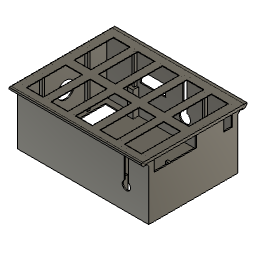
matek_enclosure (Autodesk Fusion 360 design; units mm, degrees)
Autodesk Fusion 360 part; units mm, degrees
note: some values were not read from the file. Set by a fixed rule: which sketch regions a step uses.
sketch "Sketch1" plane through (0, 0, 0) normal (0, 0, 1) x (1, 0, 0)
  line L0 (0, 0) -> (44, 0)
  line L1 (44, 0) -> (44, 29)
  line L2 (44, 29) -> (0, 29)
  line L3 (0, 29) -> (0, 0)
  line L4 (45, -1) -> (45, 30)
  line L5 (45, 30) -> (-1, 30)
  line L6 (-1, 30) -> (-1, -1)
  line L7 (-1, -1) -> (45, -1)
  line L8 (45.4, -1.4) -> (45.4, 30.4)
  line L9 (45.4, 30.4) -> (-1.4, 30.4)
  line L10 (-1.4, 30.4) -> (-1.4, -1.4)
  line L11 (-1.4, -1.4) -> (45.4, -1.4)
  line L12 (9, 30) -> (9, 29)
  line L13 (-1, 23) -> (0, 23)
  line L14 (9.8, 30) -> (9.8, 29)
  line L15 (-1, 22.2) -> (0, 22.2)
  line L16 (34.2, 30) -> (34.2, 29)
  line L17 (35, 30) -> (35, 29)
  line L18 (44, 23) -> (45, 23)
  line L19 (44, 22.2) -> (45, 22.2)
  line L20 (44, 6.8) -> (45, 6.8)
  line L21 (44, 6) -> (45, 6)
  line L22 (35, 0) -> (35, -1)
  line L23 (34.2, 0) -> (34.2, -1)
  line L24 (9, 0) -> (9, -1)
  line L25 (9.8, 0) -> (9.8, -1)
  line L26 (-1, 6.8) -> (0, 6.8)
  line L27 (-1, 6) -> (0, 6)
  line L28 (33.6, 30) -> (35.6, 30)
  line L29 (35.6, 30) -> (35.6, 28)
  line L30 (35.6, 28) -> (33.6, 28)
  line L31 (33.6, 28) -> (33.6, 30)
  line L32 (8.4, 30) -> (10.4, 30)
  line L33 (10.4, 30) -> (10.4, 28)
  line L34 (10.4, 28) -> (8.4, 28)
  line L35 (8.4, 28) -> (8.4, 30)
  line L36 (33.6, -1) -> (35.6, -1)
  line L37 (35.6, -1) -> (35.6, 1)
  line L38 (35.6, 1) -> (33.6, 1)
  line L39 (33.6, 1) -> (33.6, -1)
  line L40 (8.4, -1) -> (10.4, -1)
  line L41 (10.4, -1) -> (10.4, 1)
  line L42 (10.4, 1) -> (8.4, 1)
  line L43 (8.4, 1) -> (8.4, -1)
  dimension "d1" = 29
  dimension "d2" = 44
  dimension "d3" = 1
  dimension "d4" = 1.4
  dimension "d5" = 9
  dimension "d6" = 0.8
  dimension "d7" = 9
  dimension "d8" = 0.8
  dimension "d9" = 6
  dimension "d10" = 0.8
  dimension "d11" = 6
  dimension "d12" = 0.8
  dimension "d13" = 9
  dimension "d14" = 0.8
  dimension "d15" = 6
  dimension "d16" = 0.8
  dimension "d17" = 6
  dimension "d18" = 0.8
  dimension "d19" = 9
  dimension "d20" = 0.8
  dimension "d64" = 2
  dimension "d65" = 2
  dimension "d66" = 0.6
  dimension "d67" = 2
  dimension "d68" = 2
  dimension "d69" = 0.6
  dimension "d70" = 2
  dimension "d71" = 2
  dimension "d72" = 0.6
  dimension "d73" = 2
  dimension "d74" = 2
  dimension "d75" = 0.6
  constraint horizontal L0
  constraint vertical L1
  constraint horizontal L2
  constraint vertical L3
  constraint coincident L0.start L3.end
  constraint coincident L5 L12.start
  constraint coincident L2 L12.end
  constraint perpendicular L2 L12
  constraint coincident L6 L13.start
  constraint coincident L3 L13.end
  constraint perpendicular L3 L13
  constraint coincident L5 L14.start
  constraint coincident L2 L14.end
  constraint perpendicular L2 L14
  constraint coincident L6 L15.start
  constraint coincident L3 L15.end
  constraint perpendicular L3 L15
  constraint coincident L5 L16.start
  constraint coincident L2 L16.end
  constraint perpendicular L2 L16
  constraint coincident L5 L17.start
  constraint coincident L2 L17.end
  constraint perpendicular L2 L17
  constraint coincident L1 L18.start
  constraint coincident L4 L18.end
  constraint perpendicular L4 L18
  constraint coincident L1 L19.start
  constraint coincident L4 L19.end
  constraint perpendicular L4 L19
  constraint coincident L1 L20.start
  constraint coincident L4 L20.end
  constraint perpendicular L4 L20
  constraint coincident L1 L21.start
  constraint coincident L4 L21.end
  constraint perpendicular L4 L21
  constraint coincident L0 L22.start
  constraint coincident L7 L22.end
  constraint perpendicular L7 L22
  constraint coincident L0 L23.start
  constraint coincident L7 L23.end
  constraint perpendicular L7 L23
  constraint coincident L0 L24.start
  constraint coincident L7 L24.end
  constraint perpendicular L7 L24
  constraint coincident L0 L25.start
  constraint coincident L7 L25.end
  constraint perpendicular L7 L25
  constraint coincident L6 L26.start
  constraint coincident L3 L26.end
  constraint perpendicular L3 L26
  constraint coincident L6 L27.start
  constraint coincident L3 L27.end
  constraint perpendicular L3 L27
  constraint horizontal L28
  constraint vertical L29
  constraint horizontal L30
  constraint vertical L31
  constraint coincident L5 L28.start
  constraint horizontal L32
  constraint vertical L33
  constraint horizontal L34
  constraint vertical L35
  constraint coincident L5 L32.start
  constraint horizontal L36
  constraint vertical L37
  constraint horizontal L38
  constraint vertical L39
  constraint coincident L7 L36.start
  constraint horizontal L40
  constraint vertical L41
  constraint horizontal L42
  constraint vertical L43
  constraint coincident L7 L40.start
  measures "d1" distance of L0.start L2.end
  measures "d2" distance of L1.end L2.end
  measures "d5" distance of L3 L12
  measures "d6" distance of L12 L14
  measures "d7" distance of L1 L17
  measures "d8" distance of L16 L17.start
  measures "d9" distance of L2 L18
  measures "d10" distance of L18 L19
  measures "d11" distance of L0 L21
  measures "d12" distance of L20 L21
  measures "d13" distance of L1 L22
  measures "d14" distance of L22 L23
  measures "d15" distance of L2 L13
  measures "d16" distance of L13 L15
  measures "d17" distance of L0 L27
  measures "d18" distance of L26 L27
  measures "d19" distance of L3 L24
  measures "d20" distance of L24 L25
  measures "d64" distance of L28.end L29.end
  measures "d65" distance of L29.end L30.end
  measures "d66" distance of L17 L29
  measures "d67" distance of L33.end L34.end
  measures "d68" distance of L32.end L33.end
  measures "d69" distance of L14 L33
  measures "d70" distance of L37.end L38.end
  measures "d71" distance of L36.start L38.end
  measures "d72" distance of L23 L39
  measures "d73" distance of L41.end L42.end
  measures "d74" distance of L40.end L41.end
  measures "d75" distance of L24 L43
extrude "Extrude1" add sketch "Sketch1" along normal blind 19.8 makes body 1
extrude "Extrude2" add sketch "Sketch1" against normal blind 0.4 contours L0 L41 L42 L43 | L0 L7 L24 L40 L43 | L0 L7 L24 L25 L40 | L0 L7 L25 L40 L41 | L0 L3 L6 L7 L27 L43 | L0 L1 L2 L3 L29 L30 L31 L33 L34 L35 L37 L38 L39 L41 L42 L43 | L0 L7 L39 L41 | L0 L37 L38 L39 | L0 L7 L23 L36 L39 | L3 L6 L26 L27 | L0 L7 L22 L23 L36 | L3 L6 L15 L26 | L0 L7 L22 L36 L37 | L3 L6 L13 L15 | L0 L1 L4 L7 L21 L37 | L2 L3 L5 L6 L13 L35 | L1 L4 L20 L21 | L2 L5 L12 L32 L35 | L2 L33 L34 L35 | L1 L4 L19 L20 | L2 L5 L12 L14 L32 | L1 L4 L18 L19 | L2 L5 L14 L32 L33 | L1 L2 L4 L5 L18 L29 | L2 L5 L31 L33 | L2 L5 L16 L28 L31 | L2 L29 L30 L31 | L2 L5 L17 L28 L29 | L2 L5 L16 L17 L28 | L8 L9 L10 L11 bodies 1
extrude "Extrude3" add sketch "Sketch1" along normal up to surface (19.8 mm away) contours L0 L7 L24 L25 L40 | L3 L6 L26 L27 | L0 L7 L22 L23 L36 | L3 L6 L13 L15 | L1 L4 L20 L21 | L2 L5 L12 L14 L32 | L1 L4 L18 L19 | L2 L5 L16 L17 L28 bodies 1
sketch "Sketch2" plane through (45.4, 0, 0) normal (1, 0, 0) x (0, 1, 0)
  line L0 (30.4, -0.4) -> (30.4, 19.8)
  line L1 (30.4, 19.8) -> (-1.4, 19.8)
  line L2 (-1.4, 19.8) -> (-1.4, -0.4)
  line L3 (-1.4, -0.4) -> (30.4, -0.4)
  line L4 (-1.4, 19.8) -> (30.4, 19.8)
  line L5 (30.4, 19.8) -> (30.4, 14.8)
  line L6 (30.4, 14.8) -> (-1.4, 14.8)
  line L7 (-1.4, 14.8) -> (-1.4, 19.8)
  line L8 (15.6, 19.8) -> (15.6, 14.8)
  line L9 (25.4, 19.8) -> (25.4, 14.8)
  line L10 (0.6, 19.8) -> (0.6, 14.8)
  line L11 (28.4, 19.8) -> (28.4, 14.8)
  dimension "d27" = 5
  dimension "d28" = 17
  dimension "d29" = 5
  dimension "d30" = 2
  dimension "d31" = 2
  constraint horizontal L4
  constraint vertical L5
  constraint horizontal L6
  constraint vertical L7
  constraint coincident L0 L5.end
  constraint coincident L1.end L2.start
  constraint coincident L4 L8.start
  constraint coincident L6 L8.end
  constraint perpendicular L6 L8
  constraint coincident L1 L9.start
  constraint coincident L6 L9.end
  constraint perpendicular L6 L9
  constraint coincident L4 L10.start
  constraint coincident L6 L10.end
  constraint perpendicular L6 L10
  constraint coincident L4 L11.start
  constraint coincident L6 L11.end
  constraint perpendicular L6 L11
  measures "d27" distance of L4 L6
  measures "d28" distance of L7 L8
  measures "d29" distance of L5 L9
  measures "d30" distance of L7 L10
  measures "d31" distance of L5 L11
extrude "Extrude4" cut sketch "Sketch2" against normal blind 3 contours L1 L4 L6 L9 L11 | L1 L4 L6 L8 L10 bodies 1
sketch "Sketch4" plane through (0, -1.4, 0) normal (0, -1, 0) x (1, 0, 0)
  line L0 (45.4, -0.4) -> (45.4, 19.8)
  line L1 (45.4, 19.8) -> (-1.4, 19.8)
  line L2 (-1.4, 19.8) -> (-1.4, -0.4)
  line L3 (-1.4, -0.4) -> (45.4, -0.4)
  circle A0 centre (37.4, 7.6) radius 1.5
  line L4 (-1.4, 0) -> (45.4, 0)
  line L5 (38.15, -0.4) -> (36.65, -0.4)
  line L6 (38.15, 8.899) -> (36.65, 8.899)
  line L7 (36.65, 8.899) -> (36.65, 19.8)
  line L8 (36.65, 19.8) -> (38.15, 19.8)
  line L9 (38.15, 19.8) -> (38.15, 8.899)
  dimension "d38" = 3
  dimension "d39" = 8
  dimension "d131" = 8
  dimension "d150" = 1.5
  constraint horizontal L5
  constraint coincident L3 L5.start
  constraint horizontal L6
  constraint vertical L7
  constraint horizontal L8
  constraint vertical L9
  constraint coincident A0 L6.start
  constraint coincident A0 L6.end
  constraint collinear L1 L8
  measures "d38" diameter of A0
  measures "d39" distance of L0 A0.centre
  measures "d131" distance of L3 A0.centre
  measures "d150" distance of L7 L9
sketch "Sketch5" plane through (0, 0, 0) normal (0, 0, 1) x (1, 0, 0)
  line L0 (44, 0) -> (41, 0)
  line L1 (41, 0) -> (41, 8)
  line L2 (41, 8) -> (44, 8)
  line L3 (44, 8) -> (44, 0)
  line L4 (32.5, 8) -> (21.5, 8)
  line L5 (21.5, 8) -> (21.5, 0)
  line L6 (21.5, 0) -> (32.5, 0)
  line L7 (32.5, 0) -> (32.5, 8)
  line L8 (44, 0) -> (44, 29)
  point P0 (44, 0)
  dimension "d42" = 3
  dimension "d43" = 8
  dimension "d44" = 11.5
  dimension "d45" = 8
  dimension "d46" = 11
  constraint horizontal L0
  constraint vertical L1
  constraint horizontal L2
  constraint vertical L3
  constraint coincident P0 L0.start
  constraint horizontal L4
  constraint vertical L5
  constraint horizontal L6
  constraint vertical L7
  constraint collinear L2 L4
  measures "d42" distance of P0 L1
  measures "d43" distance of L0.end L1.end
  measures "d44" distance of L7 L8
  measures "d45" distance of L4.end L5.end
  measures "d46" distance of L4.start L4.end
extrude "Extrude7" cut sketch "Sketch5" against normal blind 2 bodies 1
sketch "Sketch8" plane through (0, 30.4, 0) normal (0, 1, 0) x (-1, 0, 0)
  line L0 (1.4, -0.4) -> (1.4, 19.8)
  line L1 (1.4, 19.8) -> (-45.4, 19.8)
  line L2 (-45.4, 19.8) -> (-45.4, -0.4)
  line L3 (-45.4, -0.4) -> (1.4, -0.4)
  line L4 (-11, 10.5) -> (-20, 10.5)
  line L5 (-20, 10.5) -> (-20, 14.5)
  line L6 (-20, 14.5) -> (-11, 14.5)
  line L7 (-11, 14.5) -> (-11, 10.5)
  line L8 (-45.4, 0) -> (1.4, 0)
  dimension "d58" = 11
  dimension "d59" = 20
  dimension "d60" = 4
  dimension "d61" = 10.5
  constraint horizontal L4
  constraint vertical L5
  constraint horizontal L6
  constraint vertical L7
  measures "d58" distance of L7 origin
  measures "d59" distance of origin L5
  measures "d60" distance of L4.end L5.end
  measures "d61" distance of L4 L8
extrude "Extrude10" cut sketch "Sketch8" against normal blind 2 contours L4 L5 L6 L7 bodies 1
sketch "Sketch9" plane through (0, 0, 0) normal (0, 0, 1) x (1, 0, 0)
extrude "Extrude11" add sketch "Sketch1" along normal blind 9 contours L0 L41 L42 L43 | L0 L7 L24 L40 L43 | L0 L7 L25 L40 L41 | L0 L37 L38 L39 | L0 L7 L23 L36 L39 | L0 L7 L22 L36 L37 | L2 L5 L12 L32 L35 | L2 L33 L34 L35 | L2 L5 L14 L32 L33 | L2 L5 L16 L28 L31 | L2 L29 L30 L31 | L2 L5 L17 L28 L29 bodies 1
extrude "Extrude6" cut sketch "Sketch4" against normal up to surface (0.4 mm away) contours L1 A0 L7 L8 L9 | A0 L6 | A0 L6 bodies 1
sketch "Sketch10" plane through (0, 0, -0.4) normal (0, 0, -1) x (1, 0, 0)
  line L0 (-1.4, 1.4) -> (-1.4, -30.4)
  line L1 (-1.4, -30.4) -> (45.4, -30.4)
  line L2 (45.4, -30.4) -> (45.4, 1.4)
  line L3 (37.4, -16) -> (43.4, -16)
  line L4 (43.4, -16) -> (43.4, -28)
  line L5 (43.4, -28) -> (37.4, -28)
  line L6 (37.4, -28) -> (37.4, -16)
  line L7 (45.4, 1.4) -> (45.4, -30.4)
  line L8 (44, 0) -> (44, -8)
  line L9 (44, -8) -> (41, -8)
  line L10 (41, -8) -> (41, 0)
  line L11 (41, 0) -> (44, 0)
  line L12 (32.5, -8) -> (21.5, -8)
  line L13 (21.5, -8) -> (21.5, 0)
  line L14 (21.5, 0) -> (32.5, 0)
  line L15 (32.5, 0) -> (32.5, -8)
  line L16 (45.4, 1.4) -> (-1.4, 1.4)
  line L17 (0.6, -28) -> (6.6, -28)
  line L18 (6.6, -28) -> (6.6, -16)
  line L19 (6.6, -16) -> (0.6, -16)
  line L20 (0.6, -16) -> (0.6, -28)
  dimension "d78" = 12
  dimension "d79" = 6
  dimension "d80" = 2
  dimension "d162" = 2.4
  dimension "d163" = 2
  dimension "d164" = 12
  dimension "d165" = 6
  dimension "d166" = 2.4
  constraint horizontal L3
  constraint vertical L4
  constraint horizontal L5
  constraint vertical L6
  constraint horizontal L17
  constraint vertical L18
  constraint horizontal L19
  constraint vertical L20
  measures "d78" distance of L3.start L5.end
  measures "d79" distance of L3.start L3.end
  measures "d80" distance of L4 L7
  measures "d162" distance of L5 L1.end
  measures "d163" distance of L0 L20
  measures "d164" distance of L17.end L18.end
  measures "d165" distance of L18.end L19.end
  measures "d166" distance of L1 L17
extrude "Extrude12" cut sketch "Sketch10" against normal blind 5 contours L3 L4 L5 L6 | L17 L18 L19 L20 bodies 1
sketch "Sketch11" plane through (-1.4, 0, 0) normal (-1, 0, 0) x (0, -1, 0)
  line L0 (1.4, 19.8) -> (-30.4, 19.8)
  line L1 (-30.4, 19.8) -> (-30.4, -0.4)
  line L2 (-30.4, -0.4) -> (1.4, -0.4)
  circle A0 centre (-15.4, 9.6) radius 3
  line L3 (-30.4, 0) -> (1.4, 0)
  line L4 (1.4, -0.4) -> (1.4, 19.8)
  dimension "d84" = 6
  dimension "d145" = 10
  dimension "d146" = 15
  measures "d84" diameter of A0
  measures "d145" distance of L2 A0.centre
  measures "d146" distance of L1 A0.centre
extrude "Extrude13" cut sketch "Sketch11" against normal blind 3 contours A0 bodies 1
sketch "Sketch14" plane through (45.4, 0, 0) normal (1, 0, 0) x (0, 1, 0)
  line L0 (25.4, 14.8) -> (25.4, 19.8)
  line L1 (25.4, 19.8) -> (15.6, 19.8)
  line L2 (15.6, 19.8) -> (15.6, 14.8)
  line L3 (15.6, 14.8) -> (0.6, 14.8)
  line L4 (-1.4, -0.4) -> (30.4, -0.4)
  line L5 (30.4, -0.4) -> (30.4, 19.8)
  line L6 (30.4, 19.8) -> (28.4, 19.8)
  line L7 (28.4, 19.8) -> (28.4, 14.8)
  line L8 (28.4, 14.8) -> (25.4, 14.8)
  line L9 (-1.4, 19.8) -> (-1.4, 17.8)
  line L10 (-1.4, 17.8) -> (-3.4, 19.8)
  line L11 (-3.4, 19.8) -> (-1.4, 19.8)
  line L12 (30.4, 19.8) -> (30.4, 17.8)
  line L13 (30.4, 17.8) -> (32.4, 19.8)
  line L14 (32.4, 19.8) -> (30.4, 19.8)
  line L15 (0.6, 14.8) -> (0.6, 19.8)
  line L16 (0.6, 19.8) -> (-1.4, 19.8)
  line L17 (-1.4, 19.8) -> (-1.4, -0.4)
  dimension "d95" = 2
  dimension "d96" = 2
  dimension "d97" = 2
  dimension "d98" = 2
  constraint perpendicular L9 L11
  constraint coincident L5.end L6.start
  constraint coincident L5 L12.end
  constraint perpendicular L6 L12
  constraint perpendicular L5 L14
  measures "d95" distance of L9.start L9.end
  measures "d96" distance of L9.start L10.end
  measures "d97" distance of L5.end L12.end
  measures "d98" distance of L5.end L13.end
extrude "Extrude16" add sketch "Sketch14" against normal up to surface (46.8 mm away) contours L5 L12 L13 L14 | L9 L10 L11 L17 bodies 1
ref_plane "WorkPlane1" through (-1.5, 14.5, 9.7) normal (-1, 0, 0) x (0, -1, 0)
sketch "Sketch15" plane through (-1.5, 14.5, 9.7) normal (-1, 0, 0) x (0, -1, 0)
  line L0 (-15.9, 10.1) -> (-15.9, 8.1)
  line L1 (-15.9, 8.1) -> (-17.9, 10.1)
  line L2 (-17.9, 10.1) -> (-15.9, 10.1)
  line L3 (15.9, 10.1) -> (15.9, 8.1)
  line L4 (15.9, 8.1) -> (17.9, 10.1)
  line L5 (17.9, 10.1) -> (15.9, 10.1)
  line L6 (16.9414, 9) -> (18.0414, 10.1)
  line L7 (18.8414, 9.7686) -> (18.8414, 10.1)
  line L8 (18.8414, 10.1) -> (18.0414, 10.1)
  line L9 (-16.9414, 9) -> (-18.0414, 10.1)
  line L10 (-18.0414, 10.1) -> (-18.8414, 10.1)
  line L11 (-18.8414, 10.1) -> (-18.8414, 9.7686)
  line L12 (18.8414, 10.1) -> (18.8414, 10.4)
  line L13 (18.8414, 10.4) -> (-18.8414, 10.4)
  line L14 (-18.8414, 10.4) -> (-18.8414, 10.1)
  line L15 (18.0414, 10.1) -> (18.0414, 10.2)
  line L16 (18.0414, 10.2) -> (-18.0414, 10.2)
  line L17 (-18.0414, 10.1) -> (-18.0414, 10.2)
  line L18 (16.9414, 9) -> (18.0728, 9)
  line L19 (18.0728, 9) -> (18.8414, 9.7686)
  line L20 (-16.9414, 9) -> (-18.0728, 9)
  line L21 (-18.0728, 9) -> (-18.8414, 9.7686)
  dimension "d103" = 0.8
  dimension "d104" = 0.1
  dimension "d105" = 0.1
  dimension "d106" = 0.8
  dimension "d107" = 0.1
  dimension "d109" = 0.2
  dimension "d116" = 1.2
  dimension "d117" = 0.8
  dimension "d118" = 0.8
  constraint perpendicular L7 L8
  constraint parallel L1 L9
  constraint parallel L2 L10
  constraint perpendicular L2 L11
  constraint parallel L4 L6
  constraint collinear L5 L8
  constraint collinear L2 L10
  constraint perpendicular L8 L12
  constraint perpendicular L10 L14
  constraint perpendicular L8 L15
  constraint horizontal L16
  constraint perpendicular L16 L17
  constraint parallel L13 L16
  constraint horizontal L18
  constraint parallel L6 L19
  constraint parallel L13 L20
  constraint parallel L9 L21
  constraint collinear L18 L20
  measures "d103" distance of L6.end L7.end
  measures "d104" distance of L4 L6
  measures "d105" distance of L1 L9
  measures "d106" distance of L9.end L11
  measures "d107" distance of L8 L16
  measures "d109" distance of L13 L16
  measures "d116" distance of L16 L18
  measures "d117" distance of L6 L19
  measures "d118" distance of L9 L21
extrude "Extrude17" add sketch "Sketch15" against normal blind 47 separate body contours L6 L7 L8 L18 L19 | L8 L10 L12 L13 L14 L15 L16 L17 | L9 L10 L11 L20 L21 makes body 2
sketch "Sketch16" plane through (45.5, 0, 0) normal (1, 0, 0) x (0, 1, 0)
  line L0 (-2.4414, 18.7) -> (-3.5414, 19.8)
  line L1 (-3.5414, 19.8) -> (-3.5414, 19.9)
  line L2 (-3.5414, 19.9) -> (32.5414, 19.9)
  line L3 (32.5414, 19.9) -> (32.5414, 19.8)
  line L4 (32.5414, 19.8) -> (31.4414, 18.7)
  line L5 (33.3414, 19.4686) -> (33.3414, 20.1)
  line L6 (33.3414, 20.1) -> (-4.3414, 20.1)
  line L7 (-4.3414, 20.1) -> (-4.3414, 19.4686)
  line L8 (32.5414, 19.8) -> (31.4414, 18.7)
  line L9 (33.3414, 19.4686) -> (33.3414, 20.1)
  line L10 (33.3414, 20.1) -> (-4.3414, 20.1)
  line L11 (-3.5728, 18.7) -> (-2.4414, 18.7)
  line L12 (-4.3414, 19.4686) -> (-3.5728, 18.7)
  line L13 (31.4414, 18.7) -> (32.5728, 18.7)
  line L14 (32.5728, 18.7) -> (33.3414, 19.4686)
  line L15 (32.9571, 19.0843) -> (-3.9571, 19.0843)
  constraint midpoint L14 L15.start
  constraint midpoint L12 L15.end
extrude "Extrude18" add sketch "Sketch16" along normal blind 0.2 bodies 2
sketch "Sketch17" plane through (0, 0, 20.1) normal (0, 0, 1) x (-1, 0, 0)
  line L0 (1.5, -33.3414) -> (1.5, 4.3414)
  line L1 (1.5, 4.3414) -> (-45.7, 4.3414)
  line L2 (-45.7, 4.3414) -> (-45.7, -33.3414)
  line L3 (-45.7, -33.3414) -> (1.5, -33.3414)
  line L4 (-42.7, 1.3414) -> (-36.7, 1.3414)
  line L5 (-36.7, 1.3414) -> (-36.7, -12.6586)
  line L6 (-36.7, -12.6586) -> (-42.7, -12.6586)
  line L7 (-42.7, -12.6586) -> (-42.7, 1.3414)
  dimension "d121" = 3
  dimension "d122" = 3
  dimension "d123" = 6
  dimension "d124" = 14
  constraint horizontal L4
  constraint vertical L5
  constraint horizontal L6
  constraint vertical L7
  measures "d121" distance of L1 L4
  measures "d122" distance of L2 L7
  measures "d123" distance of L5 L7
  measures "d124" distance of L4 L6
extrude "Extrude19" cut sketch "Sketch17" against normal up to surface (0.2 mm away) contours L4 L5 L6 L7 bodies 2
pattern_linear "R-Pattern1" count 5 spacing 8.75 along (-1, 0, 0) count 2 spacing 17 along (0, 1, 0) of "Extrude19"
sketch "Sketch21" plane through (0, 30.4, 0) normal (0, 1, 0) x (-1, 0, 0)
  line L0 (1.4, 17.8) -> (-45.4, 17.8)
  line L1 (-45.4, 17.8) -> (-45.4, -0.4)
  line L2 (-45.4, -0.4) -> (1.4, -0.4)
  line L3 (1.4, -0.4) -> (1.4, 17.8)
  line L4 (-20, 10.5) -> (-20, 14.5)
  line L5 (-20, 14.5) -> (-11, 14.5)
  line L6 (-11, 14.5) -> (-11, 10.5)
  line L7 (-11, 10.5) -> (-20, 10.5)
  circle A0 centre (-26.9, 7.6) radius 2
  line L8 (-26.15, 9.454) -> (-27.65, 9.454)
  line L9 (-27.65, 9.454) -> (-27.65, 19.8)
  line L10 (-27.65, 19.8) -> (-26.15, 19.8)
  line L11 (-26.15, 19.8) -> (-26.15, 9.454)
  line L12 (-9.8, 19.8) -> (-34.2, 19.8)
  dimension "d152" = 18.5
  dimension "d153" = 8
  dimension "d154" = 4
  dimension "d155" = 1.5
  constraint horizontal L8
  constraint vertical L9
  constraint horizontal L10
  constraint vertical L11
  constraint coincident A0 L8.start
  constraint coincident A0 L8.end
  constraint collinear L10 L12
  measures "d152" distance of L1 A0.centre
  measures "d153" distance of L2 A0.centre
  measures "d154" diameter of A0
  measures "d155" distance of L9 L11
extrude "Extrude23" cut sketch "Sketch21" along normal blind 5 and the other way blind 4 contours L0 A0 L9 L11 | L0 L9 L10 L11 L12 | A0 L8 | A0 L8 bodies 1
extrude "Extrude24" cut sketch "Sketch4" along normal blind 8 contours L1 A0 L7 L8 L9 bodies 1
named bodies: "matek_enclosure", "matek_enclosure_base"
